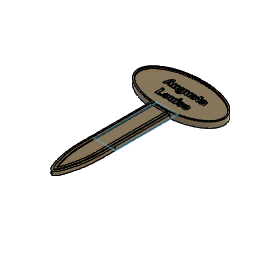
Rosen-Tafel_Augusta_Louise v5 (Autodesk Fusion 360 design; units mm, degrees)
Autodesk Fusion 360 part; units mm, degrees
sketch "Skizze1" plane through (0, 0, 0) normal (0, 0, 1) x (1, 0, 0) in component "Tafe"
  ellipse E0 centre (0, 0) end of major axis (60, 0) minor radius 30
  line L0 (-60, 0) -> (60, 0)
  line L1 (0, -30) -> (0, 30)
  dimension "d1" = 60
  constraint coincident E0.centre origin
  constraint horizontal L0
  constraint coincident E0 L0.start
  constraint coincident E0 L0.end
  constraint coincident E0 L1.start
  constraint coincident E0 L1.end
  measures "d1" distance of E0
extrude "Extrusion1" add sketch "Skizze1" along normal blind 3 makes body 1 in component "Tafe"
sketch "Skizze2" plane through (0, 0, 3) normal (0, 0, 1) x (-1, 0, 0) in component "Tafe"
  ellipse E0 centre (0, 0) end of major axis (-60, 0) minor radius 30
  spline S0 degree 3 poles (61.9509, 0) (61.9509, 4.2635) (60.3055, 8.4828) (57.3091, 12.2636) (52.6449, 18.1488) (44.7166, 23.0684) (34.8255, 26.4973) (25.2136, 29.8294) (13.7584, 31.7256) (2.1658, 31.9316) (-9.8896, 32.1459) (-22.0459, 30.5274) (-32.3487, 27.3124) (-41.3637, 24.4992) (-48.9522, 20.4892) (-54.1681, 15.6411) (-58.1005, 11.9859) (-60.7028, 7.8251) (-61.5993, 3.4465) (-62.4053, -0.4903) (-61.7899, -4.5541) (-59.8722, -8.3093) (-56.3973, -15.1137) (-48.7697, -20.9418) (-38.5998, -25.0786) (-29.6788, -28.7075) (-18.796, -31.0188) (-7.5068, -31.7189) (4.0223, -32.434) (15.9353, -31.462) (26.4461, -28.9362) (36.7725, -26.4548) (45.7187, -22.4959) (52.0049, -17.4981) (56.4978, -13.926) (59.6597, -9.8063) (61.0885, -5.3839) (61.6588, -3.6187) (61.9509, -1.8099) (61.9509, 0) knots -3.141593 -3.141593 -3.141593 -3.141593 -2.764311 -2.764311 -2.764311 -2.177028 -2.177028 -2.177028 -1.606323 -1.606323 -1.606323 -1.012833 -1.012833 -1.012833 -0.49353 -0.49353 -0.49353 -0.102016 -0.102016 -0.102016 0.249996 0.249996 0.249996 0.887852 0.887852 0.887852 1.447382 1.447382 1.447382 2.018805 2.018805 2.018805 2.580199 2.580199 2.580199 2.981436 2.981436 2.981436 3.141593 3.141593 3.141593 3.141593
  dimension "d4" = 1.9509
extrude "Extrusion2" add sketch "Skizze2" along normal blind 2 and the other way blind 2 bodies 1 in component "Tafe"
sketch "Skizze3" plane through (0, 0, 0) normal (0, 0, 1) x (1, 0, 0) in component "Tafe"
extrude "Extrusion3" add 1 faces at (23.0091, -28.1834, 1) along direction (0, 0, -1) blind 1 on bodies 1 bodies 1 in component "Tafe"
sketch "Skizze1 (2)" plane through (0, 0, 0) normal (0, 0, 1) x (1, 0, 0) in component "Ständer"
extrude "Extrusion4" add 2 faces at (23.0091, -28.1834, 0) (8.4972, -9.7981, 0) along direction (0, 0, -1) blind 3 on bodies 1 bodies 1 in component "Tafe"
sketch "Skizze2 (2)" plane through (0, 0, -3) normal (0, 0, -1) x (1, 0, 0) in component "Ständer"
  spline S0 degree 3 poles (-61.9509, 0) (-61.9509, -1.8099) (-61.6588, -3.6187) (-61.0885, -5.3839) (-59.6597, -9.8063) (-56.4978, -13.926) (-52.0049, -17.4981) (-45.7187, -22.4959) (-36.7725, -26.4548) (-26.4461, -28.9362) (-15.9353, -31.462) (-4.0223, -32.434) (7.5068, -31.7189) (18.796, -31.0188) (29.6788, -28.7075) (38.5998, -25.0786) (48.7697, -20.9418) (56.3973, -15.1137) (59.8722, -8.3093) (61.7899, -4.5541) (62.4053, -0.4903) (61.5993, 3.4465) (60.7028, 7.8251) (58.1005, 11.9859) (54.1681, 15.6411) (48.9522, 20.4892) (41.3637, 24.4992) (32.3487, 27.3124) (22.0459, 30.5274) (9.8896, 32.1459) (-2.1658, 31.9316) (-13.7584, 31.7256) (-25.2136, 29.8294) (-34.8255, 26.4973) (-44.7166, 23.0684) (-52.6449, 18.1488) (-57.3091, 12.2636) (-60.3055, 8.4828) (-61.9509, 4.2635) (-61.9509, 0) knots -3.141593 -3.141593 -3.141593 -3.141593 -2.981436 -2.981436 -2.981436 -2.580199 -2.580199 -2.580199 -2.018805 -2.018805 -2.018805 -1.447382 -1.447382 -1.447382 -0.887852 -0.887852 -0.887852 -0.249996 -0.249996 -0.249996 0.102016 0.102016 0.102016 0.49353 0.49353 0.49353 1.012833 1.012833 1.012833 1.606323 1.606323 1.606323 2.177028 2.177028 2.177028 2.764311 2.764311 2.764311 3.141593 3.141593 3.141593 3.141593
  line L0 (15, 20) -> (-15, 20)
  line L1 (-15, 20) -> (-15, 110)
  line L2 (-15, 110) -> (15, 110)
  line L3 (15, 110) -> (15, 20)
  constraint horizontal L0
  constraint vertical L1
  constraint horizontal L2
  constraint vertical L3
extrude "Extrusion1'" add sketch "Skizze2 (2)" against normal blind 5 separate body contours S0 L0 L1 L3 picked at (1.6815, 23.9477) makes body 2 in component "Ständer"
extrude "Extrusion2'" add sketch "Skizze2 (2)" against normal blind 5 contours S0 L1 L2 L3 bodies 2 in component "Ständer"
sketch "Skizze3 (2)" plane through (0, 0, 2) normal (0, 0, 1) x (-1, 0, 0) in component "Ständer"
  line L0 (15, 20) -> (15, 110)
  line L1 (15, 110) -> (-15, 110)
  line L2 (-15, 110) -> (-15, 20)
  line L3 (-15, 20) -> (15, 20)
  spline S0 degree 5 poles (15, 110) (15.0176, 110.8619) (15.0503, 112.5708) (15.0915, 115.0899) (15.1309, 118.3598) (15.1537, 122.2987) (15.1484, 126.0898) (15.1122, 129.7366) (15.0406, 133.2467) (14.9275, 136.6331) (14.7639, 139.9163) (14.5397, 143.1226) (14.2439, 146.2818) (13.867, 149.4242) (13.4012, 152.5784) (12.8426, 155.769) (12.1915, 159.0132) (11.4507, 162.3163) (10.6251, 165.6668) (9.72, 169.0317) (8.7408, 172.3517) (7.6913, 175.5347) (6.574, 178.4677) (5.3908, 181.0335) (4.1426, 183.1253) (2.8302, 184.6621) (1.7296, 185.4171) (0.8758, 185.7125) (0.294, 185.7893) (0, 185.7977) knots 0 0 0 0 0 0 0.04 0.08 0.12 0.16 0.2 0.24 0.28 0.32 0.36 0.4 0.44 0.48 0.52 0.56 0.6 0.64 0.68 0.72 0.76 0.8 0.84 0.88 0.92 0.96 1 1 1 1 1 1
  line L4 (0, -2.5) -> (0, -20)
  spline S1 degree 5 poles (-15, 110) (-15.0176, 110.8619) (-15.0503, 112.5708) (-15.0915, 115.0899) (-15.1309, 118.3598) (-15.1537, 122.2987) (-15.1484, 126.0898) (-15.1122, 129.7366) (-15.0406, 133.2467) (-14.9275, 136.6331) (-14.7639, 139.9163) (-14.5397, 143.1226) (-14.2439, 146.2818) (-13.867, 149.4242) (-13.4012, 152.5784) (-12.8426, 155.769) (-12.1915, 159.0132) (-11.4507, 162.3163) (-10.6251, 165.6668) (-9.72, 169.0317) (-8.7408, 172.3517) (-7.6913, 175.5347) (-6.574, 178.4677) (-5.3908, 181.0335) (-4.1426, 183.1253) (-2.8302, 184.6621) (-1.7296, 185.4171) (-0.8758, 185.7125) (-0.294, 185.7893) (0, 185.7977) knots 0 0 0 0 0 0 0.04 0.08 0.12 0.16 0.2 0.24 0.28 0.32 0.36 0.4 0.44 0.48 0.52 0.56 0.6 0.64 0.68 0.72 0.76 0.8 0.84 0.88 0.92 0.96 1 1 1 1 1 1
  line L5 (14.8117, 100.8471) -> (15.1883, 119.1529)
  line L6 (6.7737, 185.6047) -> (-6.7737, 185.9906)
  line L7 (-14.8117, 100.8471) -> (-15.1883, 119.1529)
  line L8 (-6.7737, 185.6047) -> (6.7737, 185.9906)
  point P0 (15, 134.2579)
  point P1 (13.5579, 151.4378)
  point P2 (9.54, 169.5876)
  point P3 (3.9981, 183.1652)
  point P4 (-15, 134.2579)
  point P5 (-13.5579, 151.4378)
  point P6 (-9.54, 169.5876)
  point P7 (-3.9981, 183.1652)
  constraint coincident L0.end L1.start
  constraint midpoint L0.end L5
  constraint midpoint S0.end L6
  constraint symmetric L0.end L4 L1.end
  constraint symmetric P0 L4 P4
  constraint symmetric P1 L4 P5
  constraint symmetric P2 L4 P6
  constraint symmetric P3 L4 P7
  constraint symmetric S0.end L4 S1.end
  constraint symmetric L4 L5.start L7.start
  constraint symmetric L4 L5.end L7.end
  constraint symmetric L4 L6.start L8.start
  constraint symmetric L4 L6.end L8.end
extrude "Extrusion3'" add sketch "Skizze3 (2)" against normal blind 5 contours L1 S0 S1 bodies 2 in component "Ständer"
sketch "Skizze4" plane through (0, 0, 2) normal (0, 0, 1) x (-1, 0, 0) in component "Ständer"
  line L0 (15, 20) -> (15, 110)
  spline S0 degree 5 poles (15, 110) (15.0176, 110.8619) (15.0503, 112.5708) (15.0915, 115.0899) (15.1309, 118.3598) (15.1537, 122.2987) (15.1484, 126.0898) (15.1122, 129.7366) (15.0406, 133.2467) (14.9275, 136.6331) (14.7639, 139.9163) (14.5397, 143.1226) (14.2439, 146.2818) (13.867, 149.4242) (13.4012, 152.5784) (12.8426, 155.769) (12.1915, 159.0132) (11.4507, 162.3163) (10.6251, 165.6668) (9.72, 169.0317) (8.7408, 172.3517) (7.6913, 175.5347) (6.574, 178.4677) (5.3908, 181.0335) (4.1426, 183.1253) (2.8302, 184.6621) (1.7296, 185.4171) (0.8758, 185.7125) (0.294, 185.7893) (0, 185.7977) knots 0 0 0 0 0 0 0.04 0.08 0.12 0.16 0.2 0.24 0.28 0.32 0.36 0.4 0.44 0.48 0.52 0.56 0.6 0.64 0.68 0.72 0.76 0.8 0.84 0.88 0.92 0.96 1 1 1 1 1 1
  spline S1 degree 5 poles (-15, 110) (-15.0176, 110.8619) (-15.0503, 112.5708) (-15.0915, 115.0899) (-15.1309, 118.3598) (-15.1537, 122.2987) (-15.1484, 126.0898) (-15.1122, 129.7366) (-15.0406, 133.2467) (-14.9275, 136.6331) (-14.7639, 139.9163) (-14.5397, 143.1226) (-14.2439, 146.2818) (-13.867, 149.4242) (-13.4012, 152.5784) (-12.8426, 155.769) (-12.1915, 159.0132) (-11.4507, 162.3163) (-10.6251, 165.6668) (-9.72, 169.0317) (-8.7408, 172.3517) (-7.6913, 175.5347) (-6.574, 178.4677) (-5.3908, 181.0335) (-4.1426, 183.1253) (-2.8302, 184.6621) (-1.7296, 185.4171) (-0.8758, 185.7125) (-0.294, 185.7893) (0, 185.7977) knots 0 0 0 0 0 0 0.04 0.08 0.12 0.16 0.2 0.24 0.28 0.32 0.36 0.4 0.44 0.48 0.52 0.56 0.6 0.64 0.68 0.72 0.76 0.8 0.84 0.88 0.92 0.96 1 1 1 1 1 1
  line L1 (-15, 110) -> (-15, 20)
  line L2 (-15, 20) -> (15, 20)
  spline S2 degree 3 poles (-11.9777, 110.0309) (-11.9779, 110.0412) (-11.9781, 110.0515) (-11.9783, 110.0618) (-12.1467, 118.2962) (-12.1876, 125.6884) (-12.0304, 132.2915) (-11.8915, 138.1249) (-11.5879, 143.3276) (-10.915, 148.5264) (-10.4464, 152.1476) (-9.7926, 155.8041) (-8.949, 159.6156) (-8.1726, 163.1233) (-7.2391, 166.7794) (-6.1929, 170.2595) (-5.0109, 174.1918) (-3.6533, 177.8638) (-2.3593, 180.1318) (-1.7058, 181.2772) (-1.0734, 182.0403) (-0.6357, 182.4064) (-0.297, 182.6897) (-0.1153, 182.7456) (0, 182.7673) knots -0.000287 -0.000287 -0.000287 -0.000287 0 0 0 0.23016 0.23016 0.23016 0.433487 0.433487 0.433487 0.575116 0.575116 0.575116 0.705456 0.705456 0.705456 0.852728 0.852728 0.852728 0.927106 0.927106 0.927106 0.984664 0.984664 0.984664 0.984664
  spline S3 degree 3 poles (11.9777, 110.0309) (11.9779, 110.0412) (11.9781, 110.0515) (11.9783, 110.0618) (12.1467, 118.2962) (12.1876, 125.6884) (12.0304, 132.2915) (11.8915, 138.1249) (11.5879, 143.3276) (10.915, 148.5264) (10.4464, 152.1476) (9.7926, 155.8041) (8.949, 159.6156) (8.1726, 163.1233) (7.2391, 166.7794) (6.1929, 170.2595) (5.0109, 174.1918) (3.6533, 177.8638) (2.3593, 180.1318) (1.7058, 181.2772) (1.0734, 182.0403) (0.6357, 182.4064) (0.297, 182.6897) (0.1153, 182.7456) (0, 182.7673) knots -0.000287 -0.000287 -0.000287 -0.000287 0 0 0 0.23016 0.23016 0.23016 0.433487 0.433487 0.433487 0.575116 0.575116 0.575116 0.705456 0.705456 0.705456 0.852728 0.852728 0.852728 0.927106 0.927106 0.927106 0.984664 0.984664 0.984664 0.984664
  line L3 (11.9777, 23.0223) -> (11.9777, 110.0309)
  line L4 (-11.9777, 23.0223) -> (11.9777, 23.0223)
  line L5 (-11.9777, 110.0309) -> (-11.9777, 23.0223)
  spline S4 degree 3 poles (-9, 110.0613) (-9.0004, 110.0818) (-9.0008, 110.1022) (-9.0013, 110.1226) (-9.1708, 118.4153) (-9.2103, 125.8461) (-9.0484, 132.4316) (-8.9146, 137.8751) (-8.6346, 142.7164) (-8.0427, 147.5055) (-7.6174, 150.9474) (-7.0241, 154.4041) (-6.2475, 158.0272) (-5.5493, 161.2843) (-4.705, 164.6878) (-3.7598, 167.9778) (-2.8347, 171.1978) (-1.801, 174.2968) (-0.8034, 176.5706) (-0.5276, 177.1992) (-0.2561, 177.763) (0, 178.2439) knots -0.000569 -0.000569 -0.000569 -0.000569 0 0 0 0.232641 0.232641 0.232641 0.424939 0.424939 0.424939 0.56314 0.56314 0.56314 0.687378 0.687378 0.687378 0.80897 0.80897 0.80897 0.842587 0.842587 0.842587 0.842587
  spline S5 degree 3 poles (9, 110.0613) (9.0004, 110.0818) (9.0008, 110.1022) (9.0013, 110.1226) (9.1708, 118.4153) (9.2103, 125.8461) (9.0484, 132.4316) (8.9146, 137.8751) (8.6346, 142.7164) (8.0427, 147.5055) (7.6174, 150.9474) (7.0241, 154.4041) (6.2475, 158.0272) (5.5493, 161.2843) (4.705, 164.6878) (3.7598, 167.9778) (2.8347, 171.1978) (1.801, 174.2968) (0.8034, 176.5706) (0.5276, 177.1992) (0.2561, 177.763) (0, 178.2439) knots -0.000569 -0.000569 -0.000569 -0.000569 0 0 0 0.232641 0.232641 0.232641 0.424939 0.424939 0.424939 0.56314 0.56314 0.56314 0.687378 0.687378 0.687378 0.80897 0.80897 0.80897 0.842587 0.842587 0.842587 0.842587
  line L6 (9, 26) -> (9, 110.0613)
  line L7 (-9, 26) -> (9, 26)
  line L8 (-9, 110.0613) -> (-9, 26)
  dimension "d19" = -3.0223
  dimension "d20" = -6
extrude "Extrusion4'" add sketch "Skizze4" along normal blind 1 contours S2 S3 L3 L4 L5 bodies 2 in component "Ständer"
combine "Kombinieren1" operation add target body 1 tool bodies 2 in component "Tafe"
sketch "Skizze1 (3)" plane through (0, 0, 3) normal (0, 0, 1) x (-1, 0, 0)
  ellipse E0 centre (0, 0) end of major axis (-60, 0) minor radius 30
  line L0 (25.6757, -14.4401) -> (22.9186, -14.4401)
  line L1 (22.9186, -14.4401) -> (19.2377, -3.4401)
  line L2 (19.2377, -3.4401) -> (22.478, -3.4401)
  line L3 (22.478, -3.4401) -> (22.8901, -4.8755)
  line L4 (22.8901, -4.8755) -> (25.2067, -4.8755)
  line L5 (25.2067, -4.8755) -> (24.5245, -7.1921)
  line L6 (24.5245, -7.1921) -> (23.5155, -7.1921)
  line L7 (23.5155, -7.1921) -> (25.6757, -14.4401)
  line L8 (26.8979, -3.4401) -> (29.9677, -3.4401)
  line L9 (29.9677, -3.4401) -> (26.6421, -13.4169)
  line L10 (26.6421, -13.4169) -> (25.2919, -8.9259)
  line L11 (25.2919, -8.9259) -> (26.8979, -3.4401)
  line L12 (14.2777, -10.9866) -> (11.4922, -10.9866)
  line L13 (11.4922, -10.9866) -> (11.4922, -3.4401)
  line L14 (11.4922, -3.4401) -> (14.2777, -3.4401)
  line L15 (14.2777, -3.4401) -> (14.2777, -10.9866)
  spline S0 degree 2 poles (15.4715, -3.5254) (15.7416, -3.4117) (16.0684, -3.3407) knots 0 0 0 1 1 1
  spline S1 degree 2 poles (16.0684, -3.3407) (16.3953, -3.2696) (16.7932, -3.2696) knots 0 0 0 1 1 1
  spline S2 degree 2 poles (16.7932, -3.2696) (17.916, -3.2696) (18.4418, -3.9091) knots 0 0 0 1 1 1
  spline S3 degree 2 poles (18.4418, -3.9091) (18.9677, -4.5487) (18.9677, -5.5861) knots 0 0 0 1 1 1
  line L16 (18.9677, -5.5861) -> (18.9677, -10.9866)
  line L17 (18.9677, -10.9866) -> (16.0684, -10.9866)
  line L18 (16.0684, -10.9866) -> (16.0684, -6.922)
  spline S4 degree 2 poles (16.0684, -6.922) (16.0684, -6.1972) (15.9547, -5.9485) knots 0 0 0 1 1 1
  spline S5 degree 2 poles (15.9547, -5.9485) (15.841, -5.6998) (15.4715, -5.643) knots 0 0 0 1 1 1
  line L19 (15.4715, -5.643) -> (15.4715, -3.5254)
  line L20 (6.0064, -8.6701) -> (6.3049, -8.6843)
  spline S6 degree 2 poles (6.3049, -8.6843) (6.6175, -8.6843) (6.8947, -8.5777) knots 0 0 0 1 1 1
  spline S7 degree 2 poles (6.8947, -8.5777) (7.1718, -8.4711) (7.3708, -8.2793) knots 0 0 0 1 1 1
  spline S8 degree 2 poles (7.3708, -8.2793) (7.5697, -8.0874) (7.6905, -7.8316) knots 0 0 0 1 1 1
  spline S9 degree 2 poles (7.6905, -7.8316) (7.8113, -7.5758) (7.8113, -7.2773) knots 0 0 0 1 1 1
  spline S10 degree 2 poles (7.8113, -7.2773) (7.8113, -6.6094) (7.3637, -6.2043) knots 0 0 0 1 1 1
  spline S11 degree 2 poles (7.3637, -6.2043) (6.916, -5.7993) (6.3049, -5.7993) knots 0 0 0 1 1 1
  line L21 (6.3049, -5.7993) -> (6.0064, -5.8135)
  line L22 (6.0064, -5.8135) -> (6.0064, -3.5965)
  spline S12 degree 2 poles (6.0064, -3.5965) (6.2338, -3.5254) (6.4896, -3.4828) knots 0 0 0 1 1 1
  spline S13 degree 2 poles (6.4896, -3.4828) (6.7454, -3.4401) (7.0297, -3.4401) knots 0 0 0 1 1 1
  spline S14 degree 2 poles (7.0297, -3.4401) (7.8397, -3.4401) (8.5006, -3.7315) knots 0 0 0 1 1 1
  spline S15 degree 2 poles (8.5006, -3.7315) (9.1615, -4.0228) (9.6233, -4.5344) knots 0 0 0 1 1 1
  spline S16 degree 2 poles (9.6233, -4.5344) (10.0852, -5.0461) (10.341, -5.7567) knots 0 0 0 1 1 1
  spline S17 degree 2 poles (10.341, -5.7567) (10.5969, -6.4673) (10.5969, -7.3058) knots 0 0 0 1 1 1
  spline S18 degree 2 poles (10.5969, -7.3058) (10.5969, -8.1443) (10.3197, -8.8478) knots 0 0 0 1 1 1
  spline S19 degree 2 poles (10.3197, -8.8478) (10.0426, -9.5512) (9.5665, -10.0629) knots 0 0 0 1 1 1
  spline S20 degree 2 poles (9.5665, -10.0629) (9.0904, -10.5745) (8.4438, -10.8658) knots 0 0 0 1 1 1
  spline S21 degree 2 poles (8.4438, -10.8658) (7.7971, -11.1572) (7.0723, -11.1572) knots 0 0 0 1 1 1
  spline S22 degree 2 poles (7.0723, -11.1572) (6.7596, -11.1572) (6.4967, -11.1217) knots 0 0 0 1 1 1
  spline S23 degree 2 poles (6.4967, -11.1217) (6.2338, -11.0861) (6.0064, -11.0151) knots 0 0 0 1 1 1
  line L23 (6.0064, -11.0151) -> (6.0064, -8.6701)
  line L24 (4.77, -10.9866) -> (1.9845, -10.9866)
  line L25 (1.9845, -10.9866) -> (1.9845, -4.5629)
  spline S24 degree 2 poles (1.9845, -4.5629) (1.9845, -3.767) (2.1683, -2.9782) knots 0 0 0 1 1 1
  spline S25 degree 2 poles (2.1683, -2.9782) (2.3522, -2.1895) (2.8399, -1.5713) knots 0 0 0 1 1 1
  spline S26 degree 2 poles (2.8399, -1.5713) (3.3277, -0.9531) (4.1839, -0.5693) knots 0 0 0 1 1 1
  spline S27 degree 2 poles (4.1839, -0.5693) (5.04, -0.1856) (6.0064, -0.1856) knots 0 0 0 1 1 1
  spline S28 degree 2 poles (6.0064, -0.1856) (6.9728, -0.1856) (7.5129, -0.2851) knots 0 0 0 1 1 1
  spline S29 degree 2 poles (7.5129, -0.2851) (8.0529, -0.3846) (8.5006, -0.5267) knots 0 0 0 1 1 1
  spline S30 degree 2 poles (8.5006, -0.5267) (8.9483, -0.6688) (9.2965, -0.8109) knots 0 0 0 1 1 1
  spline S31 degree 2 poles (9.2965, -0.8109) (9.6447, -0.9531) (9.8294, -1.0383) knots 0 0 0 1 1 1
  line L26 (9.8294, -1.0383) -> (8.9483, -2.9569)
  spline S32 degree 2 poles (8.9483, -2.9569) (8.664, -2.7722) (8.3514, -2.6301) knots 0 0 0 1 1 1
  spline S33 degree 2 poles (8.3514, -2.6301) (8.0387, -2.4879) (7.6692, -2.3885) knots 0 0 0 1 1 1
  spline S34 degree 2 poles (7.6692, -2.3885) (7.2997, -2.289) (6.5607, -2.289) knots 0 0 0 1 1 1
  spline S35 degree 2 poles (6.5607, -2.289) (5.8217, -2.289) (5.3242, -2.5945) knots 0 0 0 1 1 1
  spline S36 degree 2 poles (5.3242, -2.5945) (4.8268, -2.9001) (4.77, -3.5538) knots 0 0 0 1 1 1
  line L27 (4.77, -3.5538) -> (4.77, -10.9866)
  line L28 (-3.7429, -10.9866) -> (-6.5285, -10.9866)
  line L29 (-6.5285, -10.9866) -> (-6.5285, -3.4401)
  line L30 (-6.5285, -3.4401) -> (-3.7429, -3.4401)
  line L31 (-3.7429, -3.4401) -> (-3.7429, -10.9866)
  spline S37 degree 2 poles (-2.5491, -3.5254) (-2.2791, -3.4117) (-1.9522, -3.3407) knots 0 0 0 1 1 1
  spline S38 degree 2 poles (-1.9522, -3.3407) (-1.6254, -3.2696) (-1.2274, -3.2696) knots 0 0 0 1 1 1
  spline S39 degree 2 poles (-1.2274, -3.2696) (-0.1047, -3.2696) (0.4211, -3.9091) knots 0 0 0 1 1 1
  spline S40 degree 2 poles (0.4211, -3.9091) (0.947, -4.5487) (0.947, -5.5861) knots 0 0 0 1 1 1
  line L32 (0.947, -5.5861) -> (0.947, -10.9866)
  line L33 (0.947, -10.9866) -> (-1.9522, -10.9866)
  line L34 (-1.9522, -10.9866) -> (-1.9522, -6.922)
  spline S41 degree 2 poles (-1.9522, -6.922) (-1.9522, -6.1972) (-2.0659, -5.9485) knots 0 0 0 1 1 1
  spline S42 degree 2 poles (-2.0659, -5.9485) (-2.1796, -5.6998) (-2.5491, -5.643) knots 0 0 0 1 1 1
  line L35 (-2.5491, -5.643) -> (-2.5491, -3.5254)
  spline S43 degree 2 poles (-9.7119, -6.4104) (-9.2429, -6.5383) (-8.845, -6.7444) knots 0 0 0 1 1 1
  spline S44 degree 2 poles (-8.845, -6.7444) (-8.4471, -6.9505) (-8.1557, -7.2347) knots 0 0 0 1 1 1
  spline S45 degree 2 poles (-8.1557, -7.2347) (-7.8644, -7.5189) (-7.701, -7.8885) knots 0 0 0 1 1 1
  spline S46 degree 2 poles (-7.701, -7.8885) (-7.5375, -8.258) (-7.5375, -8.727) knots 0 0 0 1 1 1
  spline S47 degree 2 poles (-7.5375, -8.727) (-7.5375, -9.3239) (-7.7933, -9.7928) knots 0 0 0 1 1 1
  spline S48 degree 2 poles (-7.7933, -9.7928) (-8.0491, -10.2618) (-8.4897, -10.5745) knots 0 0 0 1 1 1
  spline S49 degree 2 poles (-8.4897, -10.5745) (-8.9303, -10.8872) (-9.5272, -11.0506) knots 0 0 0 1 1 1
  spline S50 degree 2 poles (-9.5272, -11.0506) (-10.1241, -11.214) (-10.792, -11.214) knots 0 0 0 1 1 1
  spline S51 degree 2 poles (-10.792, -11.214) (-11.5311, -11.214) (-12.1564, -11.0648) knots 0 0 0 1 1 1
  spline S52 degree 2 poles (-12.1564, -11.0648) (-12.7817, -10.9156) (-13.2365, -10.7308) knots 0 0 0 1 1 1
  spline S53 degree 2 poles (-13.2365, -10.7308) (-13.7765, -10.5177) (-14.2029, -10.2476) knots 0 0 0 1 1 1
  line L36 (-14.2029, -10.2476) -> (-13.2649, -8.4711)
  spline S54 degree 2 poles (-13.2649, -8.4711) (-12.9665, -8.6701) (-12.6396, -8.8122) knots 0 0 0 1 1 1
  spline S55 degree 2 poles (-12.6396, -8.8122) (-12.3127, -8.9543) (-11.9858, -9.0396) knots 0 0 0 1 1 1
  spline S56 degree 2 poles (-11.9858, -9.0396) (-11.659, -9.1249) (-11.3747, -9.1675) knots 0 0 0 1 1 1
  spline S57 degree 2 poles (-11.3747, -9.1675) (-11.0905, -9.2102) (-10.8773, -9.2102) knots 0 0 0 1 1 1
  spline S58 degree 2 poles (-10.8773, -9.2102) (-10.5931, -9.2102) (-10.4723, -9.1178) knots 0 0 0 1 1 1
  spline S59 degree 2 poles (-10.4723, -9.1178) (-10.3515, -9.0254) (-10.3515, -8.9117) knots 0 0 0 1 1 1
  spline S60 degree 2 poles (-10.3515, -8.9117) (-10.3515, -8.7554) (-10.4794, -8.6133) knots 0 0 0 1 1 1
  spline S61 degree 2 poles (-10.4794, -8.6133) (-10.6073, -8.4711) (-10.9057, -8.3574) knots 0 0 0 1 1 1
  line L37 (-10.9057, -8.3574) -> (-9.7119, -6.4104)
  spline S62 degree 2 poles (-11.0194, -3.227) (-9.8398, -3.227) (-8.9445, -3.5183) knots 0 0 0 1 1 1
  spline S63 degree 2 poles (-8.9445, -3.5183) (-8.0491, -3.8096) (-7.168, -4.506) knots 0 0 0 1 1 1
  line L38 (-7.168, -4.506) -> (-8.2055, -6.2257)
  spline S64 degree 2 poles (-8.2055, -6.2257) (-8.8876, -5.7851) (-9.5627, -5.5009) knots 0 0 0 1 1 1
  spline S65 degree 2 poles (-9.5627, -5.5009) (-10.2378, -5.2166) (-10.7778, -5.2166) knots 0 0 0 1 1 1
  spline S66 degree 2 poles (-10.7778, -5.2166) (-11.0905, -5.2166) (-11.325, -5.309) knots 0 0 0 1 1 1
  spline S67 degree 2 poles (-11.325, -5.309) (-11.5595, -5.4014) (-11.5595, -5.6003) knots 0 0 0 1 1 1
  spline S68 degree 2 poles (-11.5595, -5.6003) (-11.5595, -5.6998) (-11.46, -5.7922) knots 0 0 0 1 1 1
  spline S69 degree 2 poles (-11.46, -5.7922) (-11.3605, -5.8846) (-11.2468, -5.9556) knots 0 0 0 1 1 1
  spline S70 degree 2 poles (-11.2468, -5.9556) (-11.1047, -6.0409) (-10.9342, -6.112) knots 0 0 0 1 1 1
  line L39 (-10.9342, -6.112) -> (-12.1564, -8.0732)
  spline S71 degree 2 poles (-12.1564, -8.0732) (-12.5827, -7.9595) (-12.9807, -7.789) knots 0 0 0 1 1 1
  spline S72 degree 2 poles (-12.9807, -7.789) (-13.3786, -7.6184) (-13.6842, -7.3555) knots 0 0 0 1 1 1
  spline S73 degree 2 poles (-13.6842, -7.3555) (-13.9897, -7.0926) (-14.1745, -6.7089) knots 0 0 0 1 1 1
  spline S74 degree 2 poles (-14.1745, -6.7089) (-14.3592, -6.3251) (-14.3592, -5.8135) knots 0 0 0 1 1 1
  spline S75 degree 2 poles (-14.3592, -5.8135) (-14.3592, -5.2308) (-14.1247, -4.7547) knots 0 0 0 1 1 1
  spline S76 degree 2 poles (-14.1247, -4.7547) (-13.8902, -4.2786) (-13.4568, -3.9375) knots 0 0 0 1 1 1
  spline S77 degree 2 poles (-13.4568, -3.9375) (-13.0233, -3.5965) (-12.4051, -3.4117) knots 0 0 0 1 1 1
  spline S78 degree 2 poles (-12.4051, -3.4117) (-11.7869, -3.227) (-11.0194, -3.227) knots 0 0 0 1 1 1
  spline S79 degree 2 poles (-17.969, -3.4401) (-17.0595, -3.4401) (-16.5692, -3.7244) knots 0 0 0 1 1 1
  spline S80 degree 2 poles (-16.5692, -3.7244) (-16.0789, -4.0086) (-15.8515, -4.3497) knots 0 0 0 1 1 1
  spline S81 degree 2 poles (-15.8515, -4.3497) (-15.5957, -4.7476) (-15.553, -5.2593) knots 0 0 0 1 1 1
  line L40 (-15.553, -5.2593) -> (-15.553, -8.727)
  line L41 (-15.553, -8.727) -> (-14.8851, -8.727)
  line L42 (-14.8851, -8.727) -> (-14.8851, -10.9866)
  line L43 (-14.8851, -10.9866) -> (-15.553, -10.9866)
  line L44 (-15.553, -10.9866) -> (-15.553, -13.3458)
  line L45 (-15.553, -13.3458) -> (-18.3954, -13.3458)
  line L46 (-18.3954, -13.3458) -> (-18.3954, -10.9866)
  line L47 (-18.3954, -10.9866) -> (-19.7882, -10.9866)
  line L48 (-19.7882, -10.9866) -> (-19.7882, -8.727)
  line L49 (-19.7882, -8.727) -> (-18.3954, -8.727)
  line L50 (-18.3954, -8.727) -> (-18.3954, -6.4531)
  spline S82 degree 2 poles (-18.3954, -6.4531) (-18.3954, -6.1546) (-18.502, -5.977) knots 0 0 0 1 1 1
  spline S83 degree 2 poles (-18.502, -5.977) (-18.6086, -5.7993) (-18.9781, -5.7993) knots 0 0 0 1 1 1
  line L51 (-18.9781, -5.7993) -> (-19.7882, -5.7993)
  line L52 (-19.7882, -5.7993) -> (-19.7882, -3.4401)
  line L53 (-19.7882, -3.4401) -> (-17.969, -3.4401)
  spline S84 degree 2 poles (-23.5969, -9.2244) (-22.8437, -9.1675) (-22.3747, -9.0183) knots 0 0 0 1 1 1
  spline S85 degree 2 poles (-22.3747, -9.0183) (-21.9057, -8.8691) (-21.6215, -8.7127) knots 0 0 0 1 1 1
  line L54 (-21.6215, -8.7127) -> (-20.8967, -10.4892)
  spline S86 degree 2 poles (-20.8967, -10.4892) (-21.3088, -10.6882) (-21.9413, -10.8658) knots 0 0 0 1 1 1
  spline S87 degree 2 poles (-21.9413, -10.8658) (-22.5737, -11.0435) (-23.5969, -11.1288) knots 0 0 0 1 1 1
  line L55 (-23.5969, -11.1288) -> (-23.5969, -9.2244)
  spline S88 degree 2 poles (-24.4354, -6.8368) (-23.867, -6.8226) (-23.5401, -6.5596) knots 0 0 0 1 1 1
  spline S89 degree 2 poles (-23.5401, -6.5596) (-23.2132, -6.2967) (-23.2132, -5.8419) knots 0 0 0 1 1 1
  spline S90 degree 2 poles (-23.2132, -5.8419) (-23.2132, -5.4014) (-23.5898, -5.1953) knots 0 0 0 1 1 1
  spline S91 degree 2 poles (-23.5898, -5.1953) (-23.9665, -4.9892) (-24.4354, -4.975) knots 0 0 0 1 1 1
  line L56 (-24.4354, -4.975) -> (-24.4354, -3.4259)
  spline S92 degree 2 poles (-24.4354, -3.4259) (-24.1938, -3.3549) (-23.9238, -3.3122) knots 0 0 0 1 1 1
  spline S93 degree 2 poles (-23.9238, -3.3122) (-23.6538, -3.2696) (-23.3269, -3.2696) knots 0 0 0 1 1 1
  spline S94 degree 2 poles (-23.3269, -3.2696) (-22.7016, -3.2696) (-22.1687, -3.4543) knots 0 0 0 1 1 1
  spline S95 degree 2 poles (-22.1687, -3.4543) (-21.6357, -3.6391) (-21.252, -3.9731) knots 0 0 0 1 1 1
  spline S96 degree 2 poles (-21.252, -3.9731) (-20.8683, -4.3071) (-20.648, -4.7832) knots 0 0 0 1 1 1
  spline S97 degree 2 poles (-20.648, -4.7832) (-20.4277, -5.2593) (-20.4277, -5.8419) knots 0 0 0 1 1 1
  spline S98 degree 2 poles (-20.4277, -5.8419) (-20.4277, -6.4815) (-20.6764, -6.9576) knots 0 0 0 1 1 1
  spline S99 degree 2 poles (-20.6764, -6.9576) (-20.9251, -7.4337) (-21.3515, -7.7605) knots 0 0 0 1 1 1
  spline S100 degree 2 poles (-21.3515, -7.7605) (-21.7778, -8.0874) (-22.3534, -8.2509) knots 0 0 0 1 1 1
  spline S101 degree 2 poles (-22.3534, -8.2509) (-22.929, -8.4143) (-23.5969, -8.4143) knots 0 0 0 1 1 1
  spline S102 degree 2 poles (-23.5969, -8.4143) (-23.9665, -8.4143) (-24.4354, -8.329) knots 0 0 0 1 1 1
  line L57 (-24.4354, -8.329) -> (-24.4354, -6.8368)
  spline S103 degree 2 poles (-24.8334, -11.143) (-25.6435, -11.1003) (-26.3185, -10.8943) knots 0 0 0 1 1 1
  spline S104 degree 2 poles (-26.3185, -10.8943) (-26.9936, -10.6882) (-27.4768, -10.2547) knots 0 0 0 1 1 1
  spline S105 degree 2 poles (-27.4768, -10.2547) (-27.96, -9.8213) (-28.23, -9.132) knots 0 0 0 1 1 1
  spline S106 degree 2 poles (-28.23, -9.132) (-28.5, -8.4427) (-28.5, -7.4337) knots 0 0 0 1 1 1
  line L58 (-28.5, -7.4337) -> (-28.5, -3.4401)
  line L59 (-28.5, -3.4401) -> (-25.6719, -3.4401)
  line L60 (-25.6719, -3.4401) -> (-25.6719, -8.2153)
  spline S107 degree 2 poles (-25.6719, -8.2153) (-25.6435, -8.5848) (-25.4303, -8.8051) knots 0 0 0 1 1 1
  spline S108 degree 2 poles (-25.4303, -8.8051) (-25.2171, -9.0254) (-24.8334, -9.1107) knots 0 0 0 1 1 1
  line L61 (-24.8334, -9.1107) -> (-24.8334, -11.143)
  line L62 (18.3068, 12.5767) -> (14.8249, 12.5767)
  line L63 (14.8249, 12.5767) -> (14.8249, 15.0069)
  line L64 (14.8249, 15.0069) -> (18.3068, 15.0069)
  line L65 (18.3068, 15.0069) -> (18.3068, 12.5767)
  line L66 (22.6556, 15.0069) -> (22.6556, 4.0069)
  line L67 (22.6556, 4.0069) -> (19.5574, 4.0069)
  line L68 (19.5574, 4.0069) -> (19.5574, 15.0069)
  line L69 (19.5574, 15.0069) -> (22.6556, 15.0069)
  spline S109 degree 2 poles (11.1298, 10.0043) (11.4709, 10.1749) (11.6841, 10.5088) knots 0 0 0 1 1 1
  spline S110 degree 2 poles (11.6841, 10.5088) (11.8972, 10.8428) (11.8972, 11.255) knots 0 0 0 1 1 1
  spline S111 degree 2 poles (11.8972, 11.255) (11.8972, 11.6387) (11.6841, 11.9727) knots 0 0 0 1 1 1
  spline S112 degree 2 poles (11.6841, 11.9727) (11.4709, 12.3066) (11.1298, 12.4772) knots 0 0 0 1 1 1
  line L70 (11.1298, 12.4772) -> (11.1298, 15.149)
  spline S113 degree 2 poles (11.1298, 15.149) (11.9399, 15.0495) (12.5936, 14.7084) knots 0 0 0 1 1 1
  spline S114 degree 2 poles (12.5936, 14.7084) (13.2474, 14.3674) (13.695, 13.8486) knots 0 0 0 1 1 1
  spline S115 degree 2 poles (13.695, 13.8486) (14.1427, 13.3299) (14.3843, 12.6619) knots 0 0 0 1 1 1
  spline S116 degree 2 poles (14.3843, 12.6619) (14.6259, 11.994) (14.6259, 11.255) knots 0 0 0 1 1 1
  spline S117 degree 2 poles (14.6259, 11.255) (14.6259, 10.5017) (14.3843, 9.8267) knots 0 0 0 1 1 1
  spline S118 degree 2 poles (14.3843, 9.8267) (14.1427, 9.1516) (13.6879, 8.6329) knots 0 0 0 1 1 1
  spline S119 degree 2 poles (13.6879, 8.6329) (13.2332, 8.1141) (12.5865, 7.773) knots 0 0 0 1 1 1
  spline S120 degree 2 poles (12.5865, 7.773) (11.9399, 7.432) (11.1298, 7.3325) knots 0 0 0 1 1 1
  line L71 (11.1298, 7.3325) -> (11.1298, 10.0043)
  spline S121 degree 2 poles (9.1259, 11.255) (9.1259, 10.8428) (9.332, 10.5088) knots 0 0 0 1 1 1
  spline S122 degree 2 poles (9.332, 10.5088) (9.5381, 10.1749) (9.8934, 10.0043) knots 0 0 0 1 1 1
  line L72 (9.8934, 10.0043) -> (9.8934, 7.3325)
  spline S123 degree 2 poles (9.8934, 7.3325) (9.0833, 7.432) (8.4366, 7.7802) knots 0 0 0 1 1 1
  spline S124 degree 2 poles (8.4366, 7.7802) (7.79, 8.1283) (7.3352, 8.6542) knots 0 0 0 1 1 1
  spline S125 degree 2 poles (7.3352, 8.6542) (6.8804, 9.18) (6.6388, 9.848) knots 0 0 0 1 1 1
  spline S126 degree 2 poles (6.6388, 9.848) (6.3972, 10.5159) (6.3972, 11.255) knots 0 0 0 1 1 1
  spline S127 degree 2 poles (6.3972, 11.255) (6.3972, 11.9798) (6.6317, 12.6477) knots 0 0 0 1 1 1
  spline S128 degree 2 poles (6.6317, 12.6477) (6.8662, 13.3157) (7.3139, 13.8344) knots 0 0 0 1 1 1
  spline S129 degree 2 poles (7.3139, 13.8344) (7.7616, 14.3531) (8.4153, 14.7013) knots 0 0 0 1 1 1
  spline S130 degree 2 poles (8.4153, 14.7013) (9.0691, 15.0495) (9.8934, 15.149) knots 0 0 0 1 1 1
  line L73 (9.8934, 15.149) -> (9.8934, 12.4772)
  spline S131 degree 2 poles (9.8934, 12.4772) (9.5523, 12.3066) (9.3391, 11.9727) knots 0 0 0 1 1 1
  spline S132 degree 2 poles (9.3391, 11.9727) (9.1259, 11.6387) (9.1259, 11.255) knots 0 0 0 1 1 1
  line L74 (0.9115, 7.4604) -> (-1.8741, 7.4604)
  line L75 (-1.8741, 7.4604) -> (-1.8741, 15.0069)
  line L76 (-1.8741, 15.0069) -> (0.9115, 15.0069)
  line L77 (0.9115, 15.0069) -> (0.9115, 7.4604)
  spline S133 degree 2 poles (2.1053, 14.9216) (2.3753, 15.0353) (2.7022, 15.1064) knots 0 0 0 1 1 1
  spline S134 degree 2 poles (2.7022, 15.1064) (3.029, 15.1774) (3.427, 15.1774) knots 0 0 0 1 1 1
  spline S135 degree 2 poles (3.427, 15.1774) (4.5497, 15.1774) (5.0755, 14.5379) knots 0 0 0 1 1 1
  spline S136 degree 2 poles (5.0755, 14.5379) (5.6014, 13.8984) (5.6014, 12.8609) knots 0 0 0 1 1 1
  line L78 (5.6014, 12.8609) -> (5.6014, 7.4604)
  line L79 (5.6014, 7.4604) -> (2.7022, 7.4604)
  line L80 (2.7022, 7.4604) -> (2.7022, 11.525)
  spline S137 degree 2 poles (2.7022, 11.525) (2.7022, 12.2498) (2.5885, 12.4985) knots 0 0 0 1 1 1
  spline S138 degree 2 poles (2.5885, 12.4985) (2.4748, 12.7472) (2.1053, 12.8041) knots 0 0 0 1 1 1
  line L81 (2.1053, 12.8041) -> (2.1053, 14.9216)
  line L82 (-2.9684, 7.4604) -> (-5.7966, 7.4604)
  line L83 (-5.7966, 7.4604) -> (-5.7966, 15.0069)
  line L84 (-5.7966, 15.0069) -> (-2.9684, 15.0069)
  line L85 (-2.9684, 15.0069) -> (-2.9684, 7.4604)
  line L86 (-2.9684, 6.4513) -> (-2.9684, 4.0211)
  line L87 (-2.9684, 4.0211) -> (-5.7966, 4.0211)
  line L88 (-5.7966, 4.0211) -> (-5.7966, 6.4513)
  line L89 (-5.7966, 6.4513) -> (-2.9684, 6.4513)
  spline S139 degree 2 poles (-8.9658, 12.0366) (-8.4968, 11.9087) (-8.0989, 11.7026) knots 0 0 0 1 1 1
  spline S140 degree 2 poles (-8.0989, 11.7026) (-7.701, 11.4966) (-7.4096, 11.2123) knots 0 0 0 1 1 1
  spline S141 degree 2 poles (-7.4096, 11.2123) (-7.1183, 10.9281) (-6.9548, 10.5586) knots 0 0 0 1 1 1
  spline S142 degree 2 poles (-6.9548, 10.5586) (-6.7914, 10.1891) (-6.7914, 9.7201) knots 0 0 0 1 1 1
  spline S143 degree 2 poles (-6.7914, 9.7201) (-6.7914, 9.1232) (-7.0472, 8.6542) knots 0 0 0 1 1 1
  spline S144 degree 2 poles (-7.0472, 8.6542) (-7.303, 8.1852) (-7.7436, 7.8725) knots 0 0 0 1 1 1
  spline S145 degree 2 poles (-7.7436, 7.8725) (-8.1842, 7.5599) (-8.7811, 7.3964) knots 0 0 0 1 1 1
  spline S146 degree 2 poles (-8.7811, 7.3964) (-9.378, 7.233) (-10.0459, 7.233) knots 0 0 0 1 1 1
  spline S147 degree 2 poles (-10.0459, 7.233) (-10.7849, 7.233) (-11.4103, 7.3822) knots 0 0 0 1 1 1
  spline S148 degree 2 poles (-11.4103, 7.3822) (-12.0356, 7.5314) (-12.4904, 7.7162) knots 0 0 0 1 1 1
  spline S149 degree 2 poles (-12.4904, 7.7162) (-13.0304, 7.9294) (-13.4568, 8.1994) knots 0 0 0 1 1 1
  line L90 (-13.4568, 8.1994) -> (-12.5188, 9.9759)
  spline S150 degree 2 poles (-12.5188, 9.9759) (-12.2203, 9.7769) (-11.8935, 9.6348) knots 0 0 0 1 1 1
  spline S151 degree 2 poles (-11.8935, 9.6348) (-11.5666, 9.4927) (-11.2397, 9.4074) knots 0 0 0 1 1 1
  spline S152 degree 2 poles (-11.2397, 9.4074) (-10.9128, 9.3221) (-10.6286, 9.2795) knots 0 0 0 1 1 1
  spline S153 degree 2 poles (-10.6286, 9.2795) (-10.3444, 9.2369) (-10.1312, 9.2369) knots 0 0 0 1 1 1
  spline S154 degree 2 poles (-10.1312, 9.2369) (-9.8469, 9.2369) (-9.7261, 9.3292) knots 0 0 0 1 1 1
  spline S155 degree 2 poles (-9.7261, 9.3292) (-9.6053, 9.4216) (-9.6053, 9.5353) knots 0 0 0 1 1 1
  spline S156 degree 2 poles (-9.6053, 9.5353) (-9.6053, 9.6916) (-9.7333, 9.8338) knots 0 0 0 1 1 1
  spline S157 degree 2 poles (-9.7333, 9.8338) (-9.8612, 9.9759) (-10.1596, 10.0896) knots 0 0 0 1 1 1
  line L91 (-10.1596, 10.0896) -> (-8.9658, 12.0366)
  spline S158 degree 2 poles (-10.2733, 15.2201) (-9.0937, 15.2201) (-8.1984, 14.9287) knots 0 0 0 1 1 1
  spline S159 degree 2 poles (-8.1984, 14.9287) (-7.303, 14.6374) (-6.4219, 13.941) knots 0 0 0 1 1 1
  line L92 (-6.4219, 13.941) -> (-7.4593, 12.2214)
  spline S160 degree 2 poles (-7.4593, 12.2214) (-8.1415, 12.6619) (-8.8166, 12.9462) knots 0 0 0 1 1 1
  spline S161 degree 2 poles (-8.8166, 12.9462) (-9.4916, 13.2304) (-10.0317, 13.2304) knots 0 0 0 1 1 1
  spline S162 degree 2 poles (-10.0317, 13.2304) (-10.3444, 13.2304) (-10.5789, 13.138) knots 0 0 0 1 1 1
  spline S163 degree 2 poles (-10.5789, 13.138) (-10.8134, 13.0457) (-10.8134, 12.8467) knots 0 0 0 1 1 1
  spline S164 degree 2 poles (-10.8134, 12.8467) (-10.8134, 12.7472) (-10.7139, 12.6548) knots 0 0 0 1 1 1
  spline S165 degree 2 poles (-10.7139, 12.6548) (-10.6144, 12.5625) (-10.5007, 12.4914) knots 0 0 0 1 1 1
  spline S166 degree 2 poles (-10.5007, 12.4914) (-10.3586, 12.4061) (-10.188, 12.3351) knots 0 0 0 1 1 1
  line L93 (-10.188, 12.3351) -> (-11.4103, 10.3738)
  spline S167 degree 2 poles (-11.4103, 10.3738) (-11.8366, 10.4875) (-12.2345, 10.6581) knots 0 0 0 1 1 1
  spline S168 degree 2 poles (-12.2345, 10.6581) (-12.6325, 10.8286) (-12.938, 11.0915) knots 0 0 0 1 1 1
  spline S169 degree 2 poles (-12.938, 11.0915) (-13.2436, 11.3544) (-13.4283, 11.7382) knots 0 0 0 1 1 1
  spline S170 degree 2 poles (-13.4283, 11.7382) (-13.6131, 12.1219) (-13.6131, 12.6335) knots 0 0 0 1 1 1
  spline S171 degree 2 poles (-13.6131, 12.6335) (-13.6131, 13.2162) (-13.3786, 13.6923) knots 0 0 0 1 1 1
  spline S172 degree 2 poles (-13.3786, 13.6923) (-13.1441, 14.1684) (-12.7106, 14.5095) knots 0 0 0 1 1 1
  spline S173 degree 2 poles (-12.7106, 14.5095) (-12.2772, 14.8506) (-11.659, 15.0353) knots 0 0 0 1 1 1
  spline S174 degree 2 poles (-11.659, 15.0353) (-11.0407, 15.2201) (-10.2733, 15.2201) knots 0 0 0 1 1 1
  line L94 (-17.8482, 10.6012) -> (-19.3121, 10.6012)
  spline S175 degree 2 poles (-19.3121, 10.6012) (-19.3121, 10.2885) (-19.1699, 9.9759) knots 0 0 0 1 1 1
  spline S176 degree 2 poles (-19.1699, 9.9759) (-19.0278, 9.6632) (-18.6867, 9.5069) knots 0 0 0 1 1 1
  line L95 (-18.6867, 9.5069) -> (-18.6867, 7.3183)
  spline S177 degree 2 poles (-18.6867, 7.3183) (-19.4542, 7.4035) (-20.0724, 7.7233) knots 0 0 0 1 1 1
  spline S178 degree 2 poles (-20.0724, 7.7233) (-20.6906, 8.0431) (-21.1241, 8.5618) knots 0 0 0 1 1 1
  spline S179 degree 2 poles (-21.1241, 8.5618) (-21.5575, 9.0805) (-21.792, 9.784) knots 0 0 0 1 1 1
  spline S180 degree 2 poles (-21.792, 9.784) (-22.0265, 10.4875) (-22.0265, 11.3402) knots 0 0 0 1 1 1
  spline S181 degree 2 poles (-22.0265, 11.3402) (-22.0265, 11.525) (-21.9555, 11.6955) knots 0 0 0 1 1 1
  line L96 (-21.9555, 11.6955) -> (-17.8482, 11.6955)
  line L97 (-17.8482, 11.6955) -> (-17.8482, 10.6012)
  spline S182 degree 2 poles (-17.4503, 9.5353) (-17.1234, 9.7485) (-16.9671, 10.182) knots 0 0 0 1 1 1
  spline S183 degree 2 poles (-16.9671, 10.182) (-16.8108, 10.6154) (-16.8108, 11.0844) knots 0 0 0 1 1 1
  spline S184 degree 2 poles (-16.8108, 11.0844) (-16.8108, 11.5818) (-16.9742, 12.0437) knots 0 0 0 1 1 1
  spline S185 degree 2 poles (-16.9742, 12.0437) (-17.1376, 12.5056) (-17.4503, 12.7046) knots 0 0 0 1 1 1
  line L98 (-17.4503, 12.7046) -> (-17.4503, 15.1348)
  spline S186 degree 2 poles (-17.4503, 15.1348) (-16.6544, 15.0353) (-16.0362, 14.7013) knots 0 0 0 1 1 1
  spline S187 degree 2 poles (-16.0362, 14.7013) (-15.418, 14.3674) (-14.9917, 13.8557) knots 0 0 0 1 1 1
  spline S188 degree 2 poles (-14.9917, 13.8557) (-14.5653, 13.3441) (-14.3379, 12.6761) knots 0 0 0 1 1 1
  spline S189 degree 2 poles (-14.3379, 12.6761) (-14.1105, 12.0082) (-14.1105, 11.2407) knots 0 0 0 1 1 1
  spline S190 degree 2 poles (-14.1105, 11.2407) (-14.1105, 10.4733) (-14.345, 9.8053) knots 0 0 0 1 1 1
  spline S191 degree 2 poles (-14.345, 9.8053) (-14.5795, 9.1374) (-15.0201, 8.6258) knots 0 0 0 1 1 1
  spline S192 degree 2 poles (-15.0201, 8.6258) (-15.4606, 8.1141) (-16.0718, 7.7802) knots 0 0 0 1 1 1
  spline S193 degree 2 poles (-16.0718, 7.7802) (-16.6829, 7.4462) (-17.4503, 7.3325) knots 0 0 0 1 1 1
  line L99 (-17.4503, 7.3325) -> (-17.4503, 9.5353)
  spline S194 degree 2 poles (-21.7565, 13.3725) (-21.5149, 13.8131) (-21.117, 14.1542) knots 0 0 0 1 1 1
  spline S195 degree 2 poles (-21.117, 14.1542) (-20.719, 14.4953) (-20.1364, 14.7795) knots 0 0 0 1 1 1
  spline S196 degree 2 poles (-20.1364, 14.7795) (-19.5537, 15.0637) (-18.6867, 15.149) knots 0 0 0 1 1 1
  line L100 (-18.6867, 15.149) -> (-18.6867, 12.8893)
  spline S197 degree 2 poles (-18.6867, 12.8893) (-18.971, 12.8325) (-19.1628, 12.7188) knots 0 0 0 1 1 1
  spline S198 degree 2 poles (-19.1628, 12.7188) (-19.3547, 12.6051) (-19.4968, 12.4772) knots 0 0 0 1 1 1
  spline S199 degree 2 poles (-19.4968, 12.4772) (-19.6389, 12.3493) (-19.7384, 12.1929) knots 0 0 0 1 1 1
  line L101 (-19.7384, 12.1929) -> (-21.7565, 13.3725)
extrude "Extrusion5" cut sketch "Skizze1 (3)" against normal blind 32 contours L0 L1 L2 L3 L4 L5 L6 L7 | L8 L9 L10 L11 | L12 L13 L14 L15 | S0 S1 S2 S3 L16 L17 L18 S4 S5 L19 | L20 S6 S7 S8 S9 S10 S11 L21 L22 S12 S13 S14 S15 S16 S17 S18 S19 S20 S21 S22 S23 L23 | L24 L25 S24 S25 S26 S27 S28 S29 S30 S31 L26 S32 S33 S34 S35 S36 L27 | L28 L29 L30 L31 | S37 S38 S39 S40 L32 L33 L34 S41 S42 L35 | S43 S44 S45 S46 S47 S48 S49 S50 S51 S52 S53 L36 S54 S55 S56 S57 S58 S59 S60 S61 L37 | S62 S63 L38 S64 S65 S66 S67 S68 S69 S70 L39 S71 S72 S73 S74 S75 S76 S77 S78 | S79 S80 S81 L40 L41 L42 L43 L44 L45 L46 L47 L48 L49 L50 S82 S83 L51 L52 L53 | S84 S85 L54 S86 S87 L55 | S88 S89 S90 S91 L56 S92 S93 S94 S95 S96 S97 S98 S99 S100 S101 S102 L57 | S103 S104 S105 S106 L58 L59 L60 S107 S108 L61 | L62 L63 L64 L65 | L66 L67 L68 L69 | S109 S110 S111 S112 L70 S113 S114 S115 S116 S117 S118 S119 S120 L71 | S121 S122 L72 S123 S124 S125 S126 S127 S128 S129 S130 L73 S131 S132 | L74 L75 L76 L77 | S133 S134 S135 S136 L78 L79 L80 S137 S138 L81 | L82 L83 L84 L85 | L86 L87 L88 L89 | S139 S140 S141 S142 S143 S144 S145 S146 S147 S148 S149 L90 S150 S151 S152 S153 S154 S155 S156 S157 L91 | S158 S159 L92 S160 S161 S162 S163 S164 S165 S166 L93 S167 S168 S169 S170 S171 S172 S173 S174 | L94 S175 S176 L95 S177 S178 S179 S180 S181 L96 L97 | S182 S183 S184 S185 L98 S186 S187 S188 S189 S190 S191 S192 S193 L99 | S194 S195 S196 L100 S197 S198 S199 L101 bodies 1 in component "Tafe"
component "Tafe" placed x (1, 0, 0) y (0, 1, 0) z (0, 0, 1) at (0, 0, 0)
component "Ständer" placed x (1, 0, 0) y (0, 1, 0) z (0, 0, 1) at (0, 0, 0)
named bodies: "Grundplatte"
